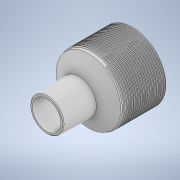
# Autodesk Inventor part: PeepBase22m
Saved by Autodesk Inventor 2020 (Build 240168000, 168)
## iProperties
Created: 2020-04-09
Part Number: PeepBase22m
Material: Generic
Document SubType Name: Modeling
Designer: Theo Cominotto
Density: 1 g/cm^3
Appearance: Default
ThreadPitch: 1,500 mm
ThreadHeight: 1,000 mm
ThreadTol: 0,100 mm
ValveD: 30,000 mm
RimT: 2,000 mm
RimH: 2,400 mm
AxleD: 2,650 mm
KnifeT: 0,200 mm
Author: Theo Cominotto
Autodesk Inventor part; units mm, degrees
ref_plane "YZ Plane" through (0, 0, 0) normal (1, 0, 0) x (0, 1, 0)
ref_plane "XY Plane" through (0, 0, 0) normal (0, 0, 1) x (1, 0, 0)
sketch "Sketch1" plane through (0, 0, 0) normal (0, 0, 1) x (1, 0, 0)
  circle A0 centre (0, 0) radius 9
  circle A1 centre (0, 0) radius 7
  dimension "d0" = 18
  dimension "d1" = 2
  constraints: 2 centre point, 1 coincident
  measures "d0" diameter of A0
  measures "d1" radial gap between concentric circles of A0 A1
extrude "Extrusion1" add sketch "Sketch1" along normal blind 2
chamfer "Chamfer1" distance 2 angle 45 1 edges at (-9, 0, 2)
sketch "Sketch4" plane through (0, 0, 0) normal (0, 1, 0) x (-1, 0, 0)
  line L0 (0, 0) -> (-12.25, 0)
  line L1 (-7, 0) -> (7, 0) projected
  line L2 (0, 0) -> (0, -8) construction
  line L3 (0, -8) -> (-18.75, -8) construction
  line L4 (-18.75, -8) -> (-12.25, 0)
  line L5 (-18.75, -8) -> (-15.75, -8)
  line L6 (-17.15, -8) -> (-11.8688, -1.5)
  line L7 (-11.8688, -1.5) -> (0, -1.5)
  line L8 (0, -1.5) -> (0, 0)
  line L9 (-7, 0) -> (-7, -1.5)
  dimension "d10" = 12.25
  dimension "d11" = 8
  dimension "d12" = 18.75
  dimension "d14" = 1.5
  dimension "d17" = 1.6
  constraints: 18 end point, 4 point on line, 3 perpendicular, 2 collinear, 1 parallel, 1 vertical
  measures "d10" distance of L0.start L0.end
  measures "d11" distance of L0.start L2.end
  measures "d12" distance of L2.end L3.end
  measures "d14" distance between parallel lines of L0 L7
  measures "d17" distance of L3.end L6.start
revolve "Revolution1" add sketch "Sketch4" angle 360 about axis through (0, 0, 0) along (0, 0, -1) contours L9 L7 L6 L5 L4 L0
sketch "Sketch5" plane through (0, 0, -8) normal (0, 0, -1) x (-1, 0, 0)
  circle A0 centre (0, 0) radius 17.15 projected
  circle A1 centre (0, 0) radius 18.75 projected
extrude "Extrusion2" add sketch "Sketch5" along normal blind 10
sketch "Sketch6" plane through (0, 0, 0) normal (0, 1, 0) x (-1, 0, 0)
  line L0 (-18.75, -18) -> (18.75, -18) construction
  line L1 (-18.75, -18) -> (-18.75, -17) construction
  line L2 (-18.75, -8) -> (-18.75, -18) construction
  line L3 (-18.75, -17) -> (-19.55, -16.4)
  line L4 (-19.55, -16.1) -> (-18.75, -15.5)
  line L5 (-19.75, -16.25) -> (-18.75, -16.25) construction
  line L6 (-19.55, -16.4) -> (-19.55, -16.1)
  line L7 (-18.69, -15.58) -> (-19.45, -16.15)
  line L8 (-19.45, -16.15) -> (-19.45, -16.35)
  line L9 (-19.45, -16.35) -> (-18.65, -16.95)
  line L10 (-18.65, -16.95) -> (-18.65, -18)
  line L11 (-18.75, -8) -> (-18.75, -18) projected
  line L12 (-18.75, -16.875) -> (-18.75, -15.625)
  line L13 (-18.75, -8) -> (-18.75, -18) projected
  point P0 (0, 0)
  dimension "d21" = 1
  dimension "d22" = 1
  dimension "d23" = 1.5
  dimension "d24" = 0.8
  dimension "d42" = 0.1
  constraints: 20 end point, 7 point on line, 1 perpendicular, 1 vertical, 4 other
  measures "d21" distance of L0.start L1.end
  measures "d22" distance of L5.start L5.end
  measures "d23" distance of L4.end L1.end
  measures "d24" distance between parallel lines of L2 L6
  measures "d42" distance between parallel lines of L3 L9
coil "Coil2" sketch "Sketch6" operation add axis through (0, 0, -10) along (0, 0, 1) pitch 1.5 turns 4 hand right contours L9 L8 L7 L11
chamfer "Chamfer4" distance 0.65 angle 45 1 edges at (19.45, 0, -10.25)
chamfer "Chamfer5" distance 0.65 angle 45 1 edges at (19.45, 0, -16.25)
sketch "Sketch8" plane through (0, 0, -18) normal (0, 0, -1) x (-1, 0, 0)
  circle A0 centre (0, 0) radius 17.15 projected
  circle A1 centre (0, 0) radius 21
  dimension "d57" = 42
  constraints: 1 centre point, 1 coincident
  measures "d57" diameter of A1
extrude "Extrusion4" add sketch "Sketch8" along normal blind 28
sketch "Sketch9" plane through (0, 0, -46) normal (0, 0, -1) x (-1, 0, 0)
  circle A0 centre (0, 0) radius 1.325
  circle A1 centre (0, 0) radius 2.525
  line L0 (0.6, 17.15) -> (-0.6, 17.15)
  line L1 (-0.6, 17.15) -> (-0.6, -17.15)
  line L2 (-0.6, -17.15) -> (0.6, -17.15)
  line L3 (0.6, -17.15) -> (0.6, 17.15)
  line L4 (0.6, 17.15) -> (-0.6, -17.15) construction
  line L5 (-0.6, 17.15) -> (0.6, -17.15) construction
  circle A2 centre (0, 0) radius 17.15 projected
  line L6 (17.15, 0.6) -> (-17.15, 0.6)
  line L7 (-17.15, 0.6) -> (-17.15, -0.6)
  line L8 (-17.15, -0.6) -> (17.15, -0.6)
  line L9 (17.15, -0.6) -> (17.15, 0.6)
  line L10 (17.15, 0.6) -> (-17.15, -0.6) construction
  line L11 (-17.15, 0.6) -> (17.15, -0.6) construction
  point P0 (-0.6, 2.4527)
  point P1 (-2.4527, 0.6)
  point P2 (-17.1395, 0.6)
  point P3 (-17.1395, -0.6)
  point P4 (-2.4527, -0.6)
  point P5 (-0.6, -2.4527)
  point P6 (-0.6, -17.1395)
  point P7 (0.6, -17.1395)
  point P8 (0.6, -2.4527)
  point P9 (2.4527, -0.6)
  point P10 (17.1395, -0.6)
  point P11 (17.1395, 0.6)
  point P12 (2.4527, 0.6)
  point P13 (0.6, 2.4527)
  point P14 (0.6, 17.1395)
  point P15 (-0.6, 17.1395)
  dimension "d60" = 2.65
  dimension "d61" = 1.2
  dimension "d62" = 1.2
  constraints: 24 end point, 4 midpoint, 4 parallel, 3 perpendicular, 2 centre point, 2 horizontal, 2 tangent, 1 coincident
  measures "d60" diameter of A0
  measures "d61" radial gap between concentric circles of A0 A1
  measures "d62" distance of L2.end L1.end
extrude "Extrusion6" add sketch "Sketch9" against normal blind 12 contours A0 L6 A1 L8 | A0 L3 A1 L6 | L8 A1 L3 A0 | A0 L1 A1 L3 | L6 A2 L8 A1 | L3 A1 L1 A0 | A0 L6 A1 L1 | A1 L1 A2 L3 | L1 A1 L8 A0 | L3 A2 L1 A1 | A0 L8 A1 L6 | A1 L8 A2 L6
sketch "Sketch10" plane through (0, 0, -46) normal (0, 0, -1) x (-1, 0, 0)
  circle A0 centre (0, 0) radius 1.325 projected
  circle A1 centre (0, 0) radius 15
  circle A2 centre (0, 0) radius 21 projected
  dimension "d67" = 30
  constraints: 1 centre point, 1 coincident
  measures "d67" diameter of A1
extrude "Extrusion7" add sketch "Sketch10" against normal blind 3 contours A2
sketch "Sketch11" plane through (0, 0, 0) normal (0, 1, 0) x (-1, 0, 0)
  line L0 (21, -18) -> (21, -46) construction
  line L1 (-21, -46) -> (21, -46) projected
  line L2 (21, -46.05) -> (21, -47.45)
  line L3 (21, -47.45) -> (22, -46.75)
  line L4 (22, -46.75) -> (21, -46.05)
  line L5 (21.65, -46.995) -> (21.65, -46.505)
  line L6 (21, -46.75) -> (22, -46.75) construction
  point P0 (0, 0)
  dimension "d74" = 1
  dimension "d75" = 0.65
  dimension "d101" = 0.75
  dimension "d102" = 1.4
  constraints: 10 end point, 2 point on line, 2 vertical, 1 collinear, 1 midpoint, 1 perpendicular, 1 other
  measures "d74" distance from line of L2 L3.end
  measures "d75" distance between parallel lines of L2 L5
  measures "d101" distance between parallel lines of L1 L6
  measures "d102" distance of L2.start L2.end
coil "Coil3" sketch "Sketch11" operation add axis through (0, 0, -10) along (0, 0, 1) pitch 1.5 turns 18.666667 hand right contours L4 L5 L3 L2
sketch "Sketch12" plane through (0, 0, -46) normal (0, 0, -1) x (0, -1, 0)
  circle A0 centre (0, 0) radius 22.5
  dimension "d84" = 45
  constraints: 1 centre point, 1 coincident
  measures "d84" diameter of A0
extrude "Extrusion8" cut sketch "Sketch12" along normal blind 20
sketch "Sketch13" plane through (0, 0, 0) normal (0, 1, 0) x (-1, 0, 0)
  line L0 (-7, 2) -> (-7, -1.5) projected
  line L1 (-7, -1.5) -> (-17.15, -11.65)
  line L2 (-17.15, -34) -> (-17.15, -8) projected
  line L3 (-7, -1.5) -> (7.3543, -1.5) construction
  line L4 (-17.15, -11.65) -> (-17.15, -8)
  line L5 (18.75, -8) -> (-18.75, -8) construction
  line L6 (11.8688, -1.5) -> (-11.8688, -1.5) projected
  line L7 (-11.8688, -1.5) -> (-17.15, -8) projected
  line L8 (0, -56.32) -> (0, 11.72) projected
  point P0 (0, 0)
  dimension "d87" = 135
  constraints: 6 end point, 3 point on line, 1 equal length, 1 horizontal, 1 vertical
  measures "d87" angle of L1 L3
revolve "Revolution2" add sketch "Sketch13" angle 360 about axis through (0, 0, -10) along (0, 0, 1)
sketch "Sketch14" plane through (0, 0, -18) normal (0, 0, 1) x (1, 0, 0)
  circle A0 centre (0, 0) radius 21 projected
  circle A1 centre (0, 0) radius 18.75 projected
  point P0 (10.5, 18.1865)
  constraints: 1 other
extrude "Extrusion9" add sketch "Sketch14" along normal blind 0.7
ref_plane "Work Plane3" through (0, 0, -17.3) normal (0, 0, 1) x (1, 0, 0)
split "Split2" plane through (0, 0, -17.3) removes the side toward (0, 0, 1)
sketch "Sketch15" plane through (0, 0, 0) normal (0, 1, 0) x (-1, 0, 0)
  line L0 (17.15, -17.3) -> (-17.15, -17.3) construction
  line L1 (0, -17.3) -> (0, -11.0781) construction
  line L2 (0, -11.0781) -> (-11.335, -11.0781) construction
  line L3 (0, -11.0781) -> (0, 9.9219) construction
  line L4 (0, 9.9219) -> (-10.81, 9.9219) construction
  line L5 (-10.81, 9.9219) -> (-11.335, -11.0781)
  line L6 (-11.335, -11.0781) -> (-21, -17.3)
  line L7 (-21, -17.3) -> (-21, -45.3) construction
  line L8 (-21, -17.3) -> (-17.15, -17.3)
  line L9 (-11.335, -11.0781) -> (-9.735, -11.0781) construction
  line L10 (-9.735, -11.0781) -> (-17.15, -17.3)
  line L11 (-10.81, 9.9219) -> (-9.21, 9.9219)
  line L12 (-9.21, 9.9219) -> (-9.735, -11.0781)
  line L13 (-11.185, -5.0781) -> (0, -5.0781) construction
  point P0 (0, 0)
  dimension "d95" = 21
  dimension "d96" = 10.81
  dimension "d97" = 1.6
  dimension "d98" = 1.6
  dimension "d99" = 40
  dimension "d157" = 15
  dimension "d158" = 11.185
  constraints: 24 end point, 5 point on line, 2 horizontal, 2 perpendicular, 2 vertical, 1 midpoint
  measures "d95" distance of L1.end L3.end
  measures "d96" distance of L3.end L4.end
  measures "d97" distance of L2.end L9.end
  measures "d98" distance of L4.end L11.end
  measures "d99" angle of L0 L10
  measures "d157" distance between parallel lines of L4 L13
  measures "d158" distance of L13.start L13.end
revolve "Revolution3" add sketch "Sketch15" angle 360 about axis through (0, 0, -11.0781) along (0, 0, 1)
ref_plane "Work Plane4" through (0, 0, 0) normal (-0.7071068, 0.7071068, 0) x (0, 0, 1)
sketch "Sketch19" plane through (0, 0, -46) normal (0, 0, -1) x (-1, 0, 0)
  circle A0 centre (0, 0) radius 5
  circle A1 centre (0, 0) radius 1.325 projected
  dimension "d120" = 10
  constraints: 1 centre point, 1 coincident
  measures "d120" diameter of A0
extrude "Extrusion10" add sketch "Sketch19" against normal blind 12
chamfer "Chamfer9" distance 0.5 angle 45 1 edges at (-10.81, 0, 9.9219)
chamfer "Chamfer10" distance 3 angle 45 4 edges at (-3.5355, -3.5355, -34) (3.5355, -3.5355, -34) (3.5355, 3.5355, -34) (-3.5355, 3.5355, -34)
chamfer "Chamfer13" distance 2.15 angle 45 4 edges at (-12.1269, -12.1269, -43) (-12.1269, 12.1269, -43) (12.1269, 12.1269, -43) (12.1269, -12.1269, -43)
sketch "Sketch20" plane through (0, 0, -46) normal (0, 0, -1) x (-1, 0, 0)
  circle A0 centre (0, 0) radius 20.7705 construction
  circle A1 centre (0, 0) radius 17 construction
  circle A2 centre (0, 0) radius 17 projected
  line L0 (0.0555, 16.9999) -> (0.0555, 20.7705) construction
  line L1 (0.0555, 18.8852) -> (0.0555, 19.6352) construction
  line L2 (0.0555, 18.8852) -> (0.0555, 18.1352) construction
  circle A3 centre (0, 0) radius 18.1353
  circle A4 centre (0, 0) radius 19.6353
  line L3 (0, 0) -> (-4.2781, 19.1636)
  line L4 (0, 0) -> (4.389, 19.1636)
  line L5 (0, 0) -> (-20.7705, 0) construction
  line L6 (0, 0) -> (-4.2781, -19.1636)
  line L7 (0, 0) -> (4.389, -19.1636)
  point P0 (-3.9513, 17.6996)
  point P1 (4.0487, 17.6776)
  point P2 (4.3836, -19.1397)
  point P3 (4.0487, -17.6776)
  point P4 (-3.9513, -17.6996)
  point P5 (4.3836, 19.1397)
  dimension "d149" = 0.75
  dimension "d150" = 0.75
  dimension "d151" = 8
  constraints: 16 end point, 7 point on circle, 4 point on line, 3 symmetric about line, 2 centre point, 2 coincident, 1 horizontal, 1 midpoint, 1 vertical, 2 other
  measures "d149" distance of L1.start L1.end
  measures "d150" distance of L1.start L2.end
  measures "d151" distance of A3.end point (4.049, 17.678)
extrude "Extrusion11" [suppressed]
equation "\"d22\" = ThreadHeight"
equation "\"d23\" = ThreadPitch"
equation "\"d42\" = ThreadTol"
equation "\"d43\" = ThreadPitch"
equation "\"d60\" = AxleD"
equation "\"d67\" = ValveD"
equation "\"d74\" = ThreadHeight"
equation "\"d101\" = 0.5 * ThreadPitch"
equation "\"d76\" = ThreadPitch"
equation "\"ThreadPitch\" = 1.5"
equation "\"ThreadHeight\" = 1"
equation "\"ThreadTol\" = 0.1"
equation "\"ValveD\" = 30"
equation "\"RimT\" = 2"
equation "\"RimH\" = 2.4"
equation "\"AxleD\" = 2.65"
equation "\"KnifeT\" = 0.2"
body "Solid1"
